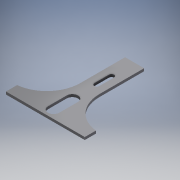
# Autodesk Inventor part: Camera stabiliser
Saved by Autodesk Inventor 2017 (Build 210142000, 142)
## iProperties
Created: 2016-08-14
Part Number: Camera stabiliser
Material: Generic
Document SubType Name: Modeling
Designer: Ali
Density: 1 g/cm^3
Appearance: Default
Author: Ali
Autodesk Inventor part; units mm, degrees
ref_plane "YZ Plane" through (0, 0, 0) normal (1, 0, 0) x (0, 1, 0)
ref_plane "XZ Plane" through (0, 0, 0) normal (0, 1, 0) x (-1, 0, 0)
ref_plane "XY Plane" through (0, 0, 0) normal (0, 0, 1) x (1, 0, 0)
sketch "Sketch1" plane through (0, 0, 0) normal (0, 0, 1) x (1, 0, 0)
  line L0 (10, -206) -> (-10, -206) construction
  line L1 (0, 0) -> (0, -45.7411)
  line L2 (-10, -206) -> (10, -206) construction
  arc A0 (-10, -160.3333) -> (10, -160.3333) centre (0, -160.3333) ccw projected
  line L3 (10, -143.6667) -> (10, -160.3333) projected
  line L4 (-10, -160.3333) -> (-10, -143.6667) projected
  arc A1 (10, -143.6667) -> (-10, -143.6667) centre (0, -143.6667) ccw projected
  circle A2 centre (-8, -187) radius 1.6 projected
  circle A3 centre (8, -187) radius 1.6 projected
  arc A4 (-5.8349, -87.227) -> (5.8349, -87.227) centre (0, -87.227) ccw projected
  line L5 (5.8349, -53.3669) -> (5.8349, -87.227) projected
  line L6 (-5.8349, -87.227) -> (-5.8349, -53.3669) projected
  arc A5 (5.8349, -53.3669) -> (-5.8349, -53.3669) centre (0, -53.3669) ccw projected
  line L7 (0, -206) -> (-90.9613, -206)
  line L8 (-90.9613, -206) -> (-90.9613, -180.2754)
  arc A6 (-90.9613, -180.2754) -> (-22, -103.3247) centre (-99.4135, -103.3247) ccw
  line L9 (-22, -103.3247) -> (-22, 74.3972)
  line L10 (0, -143.6667) -> (0, -187) construction
  line L11 (-13, -143.6667) -> (-13, -187)
  line L12 (13, -187) -> (13, -143.6667)
  arc A7 (13, -143.6667) -> (-13, -143.6667) centre (0, -143.6667) ccw
  arc A8 (-13, -187) -> (13, -187) centre (0, -187) ccw
  line L13 (0, -206) -> (90.9613, -206)
  line L14 (90.9613, -206) -> (90.9613, -180.2754)
  arc A9 (22, -103.3247) -> (90.9613, -180.2754) centre (99.4135, -103.3247) ccw
  line L15 (22, -103.3247) -> (22, 74.3972)
  line L16 (5.8349, 46.6331) -> (5.8349, 12.773) projected
  arc A10 (-5.8349, 12.773) -> (5.8349, 12.773) centre (0, 12.773) ccw projected
  line L17 (-5.8349, 12.773) -> (-5.8349, 46.6331) projected
  arc A11 (5.8349, 46.6331) -> (-5.8349, 46.6331) centre (0, 46.6331) ccw projected
  line L18 (-22, 74.3972) -> (22, 74.3972)
  point P0 (0, -165.3333)
  dimension "d2" = 26
  dimension "d5" = 22
  constraints: 24 end point, 8 point on circle, 5 symmetric about line, 5 tangent, 4 centre point, 3 midpoint, 2 perpendicular, 2 vertical, 1 collinear, 1 parallel, 1 point on line, 1 other
  measures "d2" diameter of A8
  measures "d5" distance from line of L9 L1.start
extrude "Extrusion1" add sketch "Sketch1" along normal blind 6 contours L7 L8 A6 L9 L18 L15 A9 L14 L13
body "Solid1"
